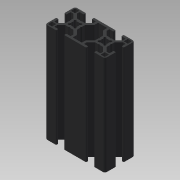
# Autodesk Inventor part: 30-3060-BLACK-FB
Saved by Autodesk Inventor 2013 (Build 170138000, 138)
## iProperties
Company: 80/20 Inc.
Created: 2014-04-23
Part Number: 30-3060-BLACK-FB
Material: Generic
Document SubType Name: Modeling
Designer: Ross Bowman
Density: 1 g/cm^3
Engineer: Ross Bowman
Catalog Web Link: 8020.net
Vendor: 80/20 Inc.
Material: 6105-T5 Aluminum
Author: Ross Bowman
Keywords: 80/20 , 8020 , T-Slot , Extrusion
Autodesk Inventor part; units mm, degrees
ref_plane "YZ Plane" through (0, 0, 0) normal (1, 0, 0) x (0, 1, 0)
ref_plane "XZ Plane" through (0, 0, 0) normal (0, 1, 0) x (-1, 0, 0)
ref_plane "XY Plane" through (0, 0, 0) normal (0, 0, 1) x (1, 0, 0)
sketch "Sketch1" plane through (0, 0, 0) normal (0, 0, 1) x (1, 0, 0)
  arc A0 (-24.5, 13.319) -> (-24.881, 13.7) centre (-24.881, 13.319) ccw
  line L0 (-24.5, 13.319) -> (-24.5, 9.88)
  arc A1 (-24.88, 9.5) -> (-24.5, 9.88) centre (-24.88, 9.88) ccw
  line L1 (-24.88, 9.5) -> (-28.3189, 9.5)
  arc A2 (-28.6999, 9.881) -> (-28.3189, 9.5) centre (-28.3189, 9.881) ccw
  line L2 (-28.6999, 9.881) -> (-28.6999, 12.7)
  arc A3 (-27.6999, 13.7) -> (-28.6999, 12.7) centre (-27.6999, 12.7) ccw
  line L3 (-27.6999, 13.7) -> (-24.881, 13.7)
  arc A4 (4.05, -12.8) -> (4.55, -12.3) centre (4.05, -12.3) ccw
  line L4 (4.05, -12.8) -> (-4.05, -12.8)
  arc A5 (-4.55, -12.3) -> (-4.05, -12.8) centre (-4.05, -12.3) ccw
  line L5 (-4.55, -12.3) -> (-4.55, -9.2682)
  arc A6 (-4.55, -9.2682) -> (-4.9893, -8.2075) centre (-6.05, -9.2682) ccw
  line L6 (-4.9893, -8.2075) -> (-9.0188, -4.178)
  arc A7 (-9.1653, -3.8245) -> (-9.0188, -4.178) centre (-8.6653, -3.8245) ccw
  line L7 (-9.1653, -3.8245) -> (-9.1653, -0.8875)
  line L8 (-9.1653, -0.8875) -> (-9.6753, 0.0625)
  line L9 (-9.6753, 0.0625) -> (-9.1653, 1.0125)
  line L10 (-9.1653, 1.0125) -> (-9.1653, 3.8245)
  arc A8 (-9.0188, 4.178) -> (-9.1653, 3.8245) centre (-8.6653, 3.8245) ccw
  line L11 (-9.0188, 4.178) -> (-4.9893, 8.2075)
  arc A9 (-4.9893, 8.2075) -> (-4.55, 9.2682) centre (-6.05, 9.2682) ccw
  line L12 (-4.55, 9.2682) -> (-4.55, 12.3)
  arc A10 (-4.05, 12.8) -> (-4.55, 12.3) centre (-4.05, 12.3) ccw
  line L13 (-4.05, 12.8) -> (4.05, 12.8)
  arc A11 (4.55, 12.3) -> (4.05, 12.8) centre (4.05, 12.3) ccw
  line L14 (4.55, 12.3) -> (4.55, 9.2682)
  arc A12 (4.55, 9.2682) -> (4.9893, 8.2075) centre (6.05, 9.2682) ccw
  line L15 (4.9893, 8.2075) -> (9.0188, 4.178)
  arc A13 (9.1653, 3.8245) -> (9.0188, 4.178) centre (8.6653, 3.8245) ccw
  line L16 (9.1653, 3.8245) -> (9.1653, 1.0125)
  line L17 (9.1653, 1.0125) -> (9.6753, 0.0625)
  line L18 (9.6753, 0.0625) -> (9.1653, -0.8875)
  line L19 (9.1653, -0.8875) -> (9.1653, -3.8245)
  arc A14 (9.0188, -4.178) -> (9.1653, -3.8245) centre (8.6653, -3.8245) ccw
  line L20 (9.0188, -4.178) -> (4.9893, -8.2075)
  arc A15 (4.9893, -8.2075) -> (4.55, -9.2682) centre (6.05, -9.2682) ccw
  line L21 (4.55, -9.2682) -> (4.55, -12.3)
  arc A16 (28.3189, 9.5) -> (28.6999, 9.881) centre (28.3189, 9.881) ccw
  line L22 (28.3189, 9.5) -> (24.88, 9.5)
  arc A17 (24.5, 9.88) -> (24.88, 9.5) centre (24.88, 9.88) ccw
  line L23 (24.5, 9.88) -> (24.5, 13.319)
  arc A18 (24.881, 13.7) -> (24.5, 13.319) centre (24.881, 13.319) ccw
  line L24 (24.881, 13.7) -> (27.6999, 13.7)
  arc A19 (28.6999, 12.7) -> (27.6999, 13.7) centre (27.6999, 12.7) ccw
  line L25 (28.6999, 12.7) -> (28.6999, 9.881)
  arc A20 (-10.9375, 13.2425) -> (-10.4375, 12.7425) centre (-10.4375, 13.2425) ccw
  line L26 (-7.2674, 12.7425) -> (-10.4375, 12.7425)
  arc A21 (-6.75, 12.2428) -> (-7.2674, 12.7425) centre (-7.25, 12.2428) ccw
  line L27 (-6.75, 10.2602) -> (-6.75, 12.2428)
  arc A22 (-6.8964, 9.9067) -> (-6.75, 10.2602) centre (-7.25, 10.2602) ccw
  line L28 (-10.822, 5.9811) -> (-6.8964, 9.9067)
  arc A23 (-11.1755, 5.8347) -> (-10.822, 5.9811) centre (-11.1755, 6.3347) ccw
  line L29 (-14.05, 5.8347) -> (-11.1755, 5.8347)
  line L30 (-15, 5.3247) -> (-14.05, 5.8347)
  line L31 (-15.95, 5.8347) -> (-15, 5.3247)
  line L32 (-18.8244, 5.8347) -> (-15.95, 5.8347)
  arc A24 (-19.178, 5.9811) -> (-18.8244, 5.8347) centre (-18.8244, 6.3347) ccw
  line L33 (-23.1035, 9.9067) -> (-19.178, 5.9811)
  arc A25 (-23.25, 10.2602) -> (-23.1035, 9.9067) centre (-22.75, 10.2602) ccw
  line L34 (-23.25, 12.2428) -> (-23.25, 10.2602)
  arc A26 (-22.7325, 12.7425) -> (-23.25, 12.2428) centre (-22.75, 12.2428) ccw
  line L35 (-19.4375, 12.7425) -> (-22.7325, 12.7425)
  arc A27 (-19.4375, 12.7425) -> (-18.9375, 13.2425) centre (-19.4375, 13.2425) ccw
  line L36 (-18.9375, 14.5) -> (-18.9375, 13.2425)
  arc A28 (-18.9375, 14.5) -> (-19.4375, 15) centre (-19.4375, 14.5) ccw
  line L37 (-27.9999, 15) -> (-19.4375, 15)
  arc A29 (-27.9999, 15) -> (-29.9999, 13) centre (-27.9999, 13) ccw
  line L38 (-29.9999, 4.5625) -> (-29.9999, 13)
  arc A30 (-29.9999, 4.5625) -> (-29.4999, 4.0625) centre (-29.4999, 4.5625) ccw
  line L39 (-28.2425, 4.0625) -> (-29.4999, 4.0625)
  arc A31 (-28.2425, 4.0625) -> (-27.7425, 4.5625) centre (-28.2425, 4.5625) ccw
  line L40 (-27.7425, 7.7325) -> (-27.7425, 4.5625)
  arc A32 (-27.2428, 8.25) -> (-27.7425, 7.7325) centre (-27.2428, 7.75) ccw
  line L41 (-25.2602, 8.25) -> (-27.2428, 8.25)
  arc A33 (-24.9066, 8.1035) -> (-25.2602, 8.25) centre (-25.2602, 7.75) ccw
  line L42 (-20.9811, 4.178) -> (-24.9066, 8.1035)
  arc A34 (-20.8347, 3.8245) -> (-20.9811, 4.178) centre (-21.3347, 3.8245) ccw
  line L43 (-20.8347, 1.0125) -> (-20.8347, 3.8245)
  line L44 (-20.3247, 0.0625) -> (-20.8347, 1.0125)
  line L45 (-20.8347, -0.8875) -> (-20.3247, 0.0625)
  line L46 (-20.8347, -3.8245) -> (-20.8347, -0.8875)
  arc A35 (-20.9811, -4.178) -> (-20.8347, -3.8245) centre (-21.3347, -3.8245) ccw
  line L47 (-24.9066, -8.1035) -> (-20.9811, -4.178)
  arc A36 (-25.2602, -8.25) -> (-24.9066, -8.1035) centre (-25.2602, -7.75) ccw
  line L48 (-27.2428, -8.25) -> (-25.2602, -8.25)
  arc A37 (-27.7425, -7.7325) -> (-27.2428, -8.25) centre (-27.2428, -7.75) ccw
  line L49 (-27.7425, -4.4375) -> (-27.7425, -7.7325)
  arc A38 (-27.7425, -4.4375) -> (-28.2425, -3.9375) centre (-28.2425, -4.4375) ccw
  line L50 (-29.4999, -3.9375) -> (-28.2425, -3.9375)
  arc A39 (-29.4999, -3.9375) -> (-29.9999, -4.4375) centre (-29.4999, -4.4375) ccw
  line L51 (-29.9999, -13) -> (-29.9999, -4.4375)
  arc A40 (-29.9999, -13) -> (-27.9999, -15) centre (-27.9999, -13) ccw
  line L52 (-19.5625, -15) -> (-27.9999, -15)
  arc A41 (-19.5625, -15) -> (-19.0625, -14.5) centre (-19.5625, -14.5) ccw
  line L53 (-19.0625, -13.2425) -> (-19.0625, -14.5)
  arc A42 (-19.0625, -13.2425) -> (-19.5625, -12.7425) centre (-19.5625, -13.2425) ccw
  line L54 (-22.7325, -12.7425) -> (-19.5625, -12.7425)
  arc A43 (-23.25, -12.2428) -> (-22.7325, -12.7425) centre (-22.75, -12.2428) ccw
  line L55 (-23.25, -10.2602) -> (-23.25, -12.2428)
  arc A44 (-23.1035, -9.9067) -> (-23.25, -10.2602) centre (-22.75, -10.2602) ccw
  line L56 (-19.178, -5.9811) -> (-23.1035, -9.9067)
  arc A45 (-18.8244, -5.8347) -> (-19.178, -5.9811) centre (-18.8244, -6.3347) ccw
  line L57 (-15.95, -5.8347) -> (-18.8244, -5.8347)
  line L58 (-15, -5.3247) -> (-15.95, -5.8347)
  line L59 (-14.05, -5.8347) -> (-15, -5.3247)
  line L60 (-11.1755, -5.8347) -> (-14.05, -5.8347)
  arc A46 (-10.822, -5.9811) -> (-11.1755, -5.8347) centre (-11.1755, -6.3347) ccw
  line L61 (-6.8964, -9.9067) -> (-10.822, -5.9811)
  arc A47 (-6.75, -10.2602) -> (-6.8964, -9.9067) centre (-7.25, -10.2602) ccw
  line L62 (-6.75, -12.2428) -> (-6.75, -10.2602)
  arc A48 (-7.2674, -12.7425) -> (-6.75, -12.2428) centre (-7.25, -12.2428) ccw
  line L63 (-10.5625, -12.7425) -> (-7.2674, -12.7425)
  arc A49 (-10.5625, -12.7425) -> (-11.0625, -13.2425) centre (-10.5625, -13.2425) ccw
  line L64 (-11.0625, -14.5) -> (-11.0625, -13.2425)
  arc A50 (-11.0625, -14.5) -> (-10.5625, -15) centre (-10.5625, -14.5) ccw
  line L65 (10.5625, -15) -> (-10.5625, -15)
  arc A51 (10.5625, -15) -> (11.0625, -14.5) centre (10.5625, -14.5) ccw
  line L66 (11.0625, -13.2425) -> (11.0625, -14.5)
  arc A52 (11.0625, -13.2425) -> (10.5625, -12.7425) centre (10.5625, -13.2425) ccw
  line L67 (7.2674, -12.7425) -> (10.5625, -12.7425)
  arc A53 (6.75, -12.2428) -> (7.2674, -12.7425) centre (7.25, -12.2428) ccw
  line L68 (6.75, -10.2602) -> (6.75, -12.2428)
  arc A54 (6.8964, -9.9067) -> (6.75, -10.2602) centre (7.25, -10.2602) ccw
  line L69 (10.822, -5.9811) -> (6.8964, -9.9067)
  arc A55 (11.1755, -5.8347) -> (10.822, -5.9811) centre (11.1755, -6.3347) ccw
  line L70 (14.05, -5.8347) -> (11.1755, -5.8347)
  line L71 (15, -5.3247) -> (14.05, -5.8347)
  line L72 (15.95, -5.8347) -> (15, -5.3247)
  line L73 (18.8244, -5.8347) -> (15.95, -5.8347)
  arc A56 (19.178, -5.9811) -> (18.8244, -5.8347) centre (18.8244, -6.3347) ccw
  line L74 (23.1035, -9.9067) -> (19.178, -5.9811)
  arc A57 (23.25, -10.2602) -> (23.1035, -9.9067) centre (22.75, -10.2602) ccw
  line L75 (23.25, -12.2428) -> (23.25, -10.2602)
  arc A58 (22.7325, -12.7425) -> (23.25, -12.2428) centre (22.75, -12.2428) ccw
  line L76 (19.5625, -12.7425) -> (22.7325, -12.7425)
  arc A59 (19.5625, -12.7425) -> (19.0625, -13.2425) centre (19.5625, -13.2425) ccw
  line L77 (19.0625, -14.5) -> (19.0625, -13.2425)
  arc A60 (19.0625, -14.5) -> (19.5625, -15) centre (19.5625, -14.5) ccw
  line L78 (27.9999, -15) -> (19.5625, -15)
  arc A61 (27.9999, -15) -> (29.9999, -13) centre (27.9999, -13) ccw
  line L79 (29.9999, -4.4375) -> (29.9999, -13)
  arc A62 (29.9999, -4.4375) -> (29.4999, -3.9375) centre (29.4999, -4.4375) ccw
  line L80 (28.2425, -3.9375) -> (29.4999, -3.9375)
  arc A63 (28.2425, -3.9375) -> (27.7425, -4.4375) centre (28.2425, -4.4375) ccw
  line L81 (27.7425, -7.7325) -> (27.7425, -4.4375)
  arc A64 (27.2428, -8.25) -> (27.7425, -7.7325) centre (27.2428, -7.75) ccw
  line L82 (25.2602, -8.25) -> (27.2428, -8.25)
  arc A65 (24.9066, -8.1035) -> (25.2602, -8.25) centre (25.2602, -7.75) ccw
  line L83 (20.9811, -4.178) -> (24.9066, -8.1035)
  arc A66 (20.8347, -3.8245) -> (20.9811, -4.178) centre (21.3347, -3.8245) ccw
  line L84 (20.8347, -0.8875) -> (20.8347, -3.8245)
  line L85 (20.3247, 0.0625) -> (20.8347, -0.8875)
  line L86 (20.8347, 1.0125) -> (20.3247, 0.0625)
  line L87 (20.8347, 3.8245) -> (20.8347, 1.0125)
  arc A67 (20.9811, 4.178) -> (20.8347, 3.8245) centre (21.3347, 3.8245) ccw
  line L88 (24.9066, 8.1035) -> (20.9811, 4.178)
  arc A68 (25.2602, 8.25) -> (24.9066, 8.1035) centre (25.2602, 7.75) ccw
  line L89 (27.2428, 8.25) -> (25.2602, 8.25)
  arc A69 (27.7425, 7.7325) -> (27.2428, 8.25) centre (27.2428, 7.75) ccw
  line L90 (27.7425, 4.5625) -> (27.7425, 7.7325)
  arc A70 (27.7425, 4.5625) -> (28.2425, 4.0625) centre (28.2425, 4.5625) ccw
  line L91 (29.4999, 4.0625) -> (28.2425, 4.0625)
  arc A71 (29.4999, 4.0625) -> (29.9999, 4.5625) centre (29.4999, 4.5625) ccw
  line L92 (29.9999, 13) -> (29.9999, 4.5625)
  arc A72 (29.9999, 13) -> (27.9999, 15) centre (27.9999, 13) ccw
  line L93 (19.4375, 15) -> (27.9999, 15)
  arc A73 (19.4375, 15) -> (18.9375, 14.5) centre (19.4375, 14.5) ccw
  line L94 (18.9375, 13.2425) -> (18.9375, 14.5)
  arc A74 (18.9375, 13.2425) -> (19.4375, 12.7425) centre (19.4375, 13.2425) ccw
  line L95 (22.7325, 12.7425) -> (19.4375, 12.7425)
  arc A75 (23.25, 12.2428) -> (22.7325, 12.7425) centre (22.75, 12.2428) ccw
  line L96 (23.25, 10.2602) -> (23.25, 12.2428)
  arc A76 (23.1035, 9.9067) -> (23.25, 10.2602) centre (22.75, 10.2602) ccw
  line L97 (19.178, 5.9811) -> (23.1035, 9.9067)
  arc A77 (18.8244, 5.8347) -> (19.178, 5.9811) centre (18.8244, 6.3347) ccw
  line L98 (15.95, 5.8347) -> (18.8244, 5.8347)
  line L99 (15, 5.3247) -> (15.95, 5.8347)
  line L100 (14.05, 5.8347) -> (15, 5.3247)
  line L101 (11.1755, 5.8347) -> (14.05, 5.8347)
  arc A78 (10.822, 5.9811) -> (11.1755, 5.8347) centre (11.1755, 6.3347) ccw
  line L102 (6.8964, 9.9067) -> (10.822, 5.9811)
  arc A79 (6.75, 10.2602) -> (6.8964, 9.9067) centre (7.25, 10.2602) ccw
  line L103 (6.75, 12.2428) -> (6.75, 10.2602)
  arc A80 (7.2674, 12.7425) -> (6.75, 12.2428) centre (7.25, 12.2428) ccw
  line L104 (10.4375, 12.7425) -> (7.2674, 12.7425)
  arc A81 (10.4375, 12.7425) -> (10.9375, 13.2425) centre (10.4375, 13.2425) ccw
  line L105 (10.9375, 14.5) -> (10.9375, 13.2425)
  arc A82 (10.9375, 14.5) -> (10.4375, 15) centre (10.4375, 14.5) ccw
  line L106 (-10.4375, 15) -> (10.4375, 15)
  arc A83 (-10.4375, 15) -> (-10.9375, 14.5) centre (-10.4375, 14.5) ccw
  line L107 (-10.9375, 13.2425) -> (-10.9375, 14.5)
  arc A84 (28.6999, -9.881) -> (28.3189, -9.5) centre (28.3189, -9.881) ccw
  line L108 (28.6999, -9.881) -> (28.6999, -12.7)
  arc A85 (27.6999, -13.7) -> (28.6999, -12.7) centre (27.6999, -12.7) ccw
  line L109 (27.6999, -13.7) -> (24.881, -13.7)
  arc A86 (24.5, -13.319) -> (24.881, -13.7) centre (24.881, -13.319) ccw
  line L110 (24.5, -13.319) -> (24.5, -9.88)
  arc A87 (24.88, -9.5) -> (24.5, -9.88) centre (24.88, -9.88) ccw
  line L111 (24.88, -9.5) -> (28.3189, -9.5)
  arc A88 (13.6606, -3.0433) -> (16.3393, -3.0433) centre (15, 0) ccw
  line L112 (13.6606, -3.0433) -> (12.6815, -3.8251)
  arc A89 (11.1749, -2.3185) -> (12.6815, -3.8251) centre (12.0126, -2.9874) ccw
  line L113 (11.1749, -2.3185) -> (11.9567, -1.3394)
  arc A90 (11.9608, 1.3486) -> (11.9567, -1.3394) centre (15, 0) ccw
  line L114 (11.9608, 1.3486) -> (11.179, 2.3278)
  arc A91 (12.6856, 3.8343) -> (11.179, 2.3278) centre (12.0167, 2.9966) ccw
  line L115 (12.6856, 3.8343) -> (13.6707, 3.0477)
  arc A92 (16.3393, 3.0433) -> (13.6707, 3.0477) centre (15, 0) ccw
  line L116 (16.3393, 3.0433) -> (17.3185, 3.8251)
  arc A93 (18.8251, 2.3185) -> (17.3185, 3.8251) centre (17.9873, 2.9874) ccw
  line L117 (18.8251, 2.3185) -> (18.0433, 1.3394)
  arc A94 (18.0433, -1.3394) -> (18.0433, 1.3394) centre (15, 0) ccw
  line L118 (18.0433, -1.3394) -> (18.8251, -2.3185)
  arc A95 (17.3185, -3.8251) -> (18.8251, -2.3185) centre (17.9873, -2.9874) ccw
  line L119 (17.3185, -3.8251) -> (16.3393, -3.0433)
  arc A96 (-16.3393, -3.0433) -> (-13.6606, -3.0433) centre (-15, 0) ccw
  line L120 (-16.3393, -3.0433) -> (-17.3185, -3.8251)
  arc A97 (-18.8251, -2.3185) -> (-17.3185, -3.8251) centre (-17.9873, -2.9874) ccw
  line L121 (-18.8251, -2.3185) -> (-18.0433, -1.3394)
  arc A98 (-18.0392, 1.3486) -> (-18.0433, -1.3394) centre (-15, 0) ccw
  line L122 (-18.0392, 1.3486) -> (-18.821, 2.3278)
  arc A99 (-17.3144, 3.8343) -> (-18.821, 2.3278) centre (-17.9833, 2.9966) ccw
  line L123 (-17.3144, 3.8343) -> (-16.3292, 3.0477)
  arc A100 (-13.6606, 3.0433) -> (-16.3292, 3.0477) centre (-15, 0) ccw
  line L124 (-13.6606, 3.0433) -> (-12.6815, 3.8251)
  arc A101 (-11.1749, 2.3185) -> (-12.6815, 3.8251) centre (-12.0126, 2.9874) ccw
  line L125 (-11.1749, 2.3185) -> (-11.9567, 1.3394)
  arc A102 (-11.9567, -1.3394) -> (-11.9567, 1.3394) centre (-15, 0) ccw
  line L126 (-11.9567, -1.3394) -> (-11.1749, -2.3185)
  arc A103 (-12.6815, -3.8251) -> (-11.1749, -2.3185) centre (-12.0126, -2.9874) ccw
  line L127 (-12.6815, -3.8251) -> (-13.6606, -3.0433)
  arc A104 (-28.3189, -9.5) -> (-28.6999, -9.881) centre (-28.3189, -9.881) ccw
  line L128 (-28.3189, -9.5) -> (-24.88, -9.5)
  arc A105 (-24.5, -9.88) -> (-24.88, -9.5) centre (-24.88, -9.88) ccw
  line L129 (-24.5, -9.88) -> (-24.5, -13.319)
  arc A106 (-24.881, -13.7) -> (-24.5, -13.319) centre (-24.881, -13.319) ccw
  line L130 (-24.881, -13.7) -> (-27.6999, -13.7)
  arc A107 (-28.6999, -12.7) -> (-27.6999, -13.7) centre (-27.6999, -12.7) ccw
  line L131 (-28.6999, -12.7) -> (-28.6999, -9.881)
  point P0 (0, 0)
  constraints: 264 end point, 216 point on circle, 108 centre point
extrude "Extrusion1" add sketch "Sketch1" against normal blind 100
body "Solid1"
